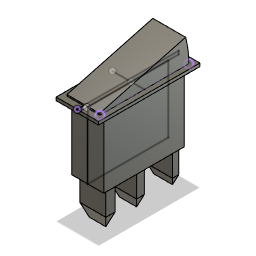
switch v2 (Autodesk Fusion 360 design; units mm, degrees)
Autodesk Fusion 360 part; units mm, degrees
sketch "Sketch1" plane through (0, 0, 0) normal (1, 0, 0) x (0, 0, -1)
  line L0 (0, 0) -> (32.5, 0)
  line L1 (32.5, 0) -> (32.5, -1)
  line L2 (32.5, -1) -> (0, -1)
  line L3 (0, -1) -> (0, 0)
  line L4 (0, -1) -> (3.35, -1) construction
  line L5 (3.35, -1) -> (29.15, -1)
  line L6 (29.15, -1) -> (29.15, -22.4)
  line L7 (29.15, -22.4) -> (3.35, -22.4)
  line L8 (3.35, -22.4) -> (3.35, -1)
  dimension "d1" = 32.5
  dimension "d2" = 1
  dimension "d3" = 3.35
  dimension "d4" = 25.8
  dimension "d5" = 21.4
  constraint horizontal L0
  constraint vertical L1
  constraint horizontal L2
  constraint vertical L3
  constraint coincident L0.start L3.end
  constraint perpendicular L3 L4
  constraint horizontal L5
  constraint vertical L6
  constraint horizontal L7
  constraint vertical L8
  measures "d1" distance of L0.start L0.end
  measures "d2" distance of L0.start L2.end
  measures "d3" distance of L2.end L4.end
  measures "d4" distance of L4.end L5.end
  measures "d5" distance of L4.end L7.end
extrude "Extrude1" add sketch "Sketch1" along normal mid plane 13.6 contours L0 L1 L2 L3 L5 makes body 1
extrude "Extrude2" add sketch "Sketch1" along normal mid plane 10.3 contours L2 L5 L6 L7 L8 bodies 1
sketch "Sketch2" plane through (0, 0, 0) normal (0, 1, 0) x (-1, 0, 0)
  line L0 (6.8, 0) -> (-6.8, 0)
  line L1 (-6.8, 0) -> (-6.8, -32.5)
  line L2 (-6.8, -32.5) -> (6.8, -32.5)
  line L3 (6.8, -32.5) -> (6.8, 0)
  line L4 (6.8, 0) -> (5.25, 0) construction
  line L5 (5.25, 0) -> (5.25, -2) construction
  line L6 (5.25, -2) -> (5.25, -30.5) construction
  line L7 (5.25, -30.5) -> (-5.25, -30.5)
  line L8 (-5.25, -30.5) -> (-5.25, -2)
  line L9 (-5.25, -2) -> (5.25, -2)
  line L10 (5.25, -2) -> (5.25, -30.5)
  dimension "d10" = 1.55
  dimension "d11" = 2
  dimension "d12" = 28.5
  dimension "d13" = 10.5
  constraint coincident L3 L0.start
  constraint perpendicular L3 L4
  constraint coincident L0 L3.end
  constraint perpendicular L0 L5
  constraint perpendicular L2 L6
  constraint horizontal L7
  constraint vertical L8
  constraint horizontal L9
  constraint vertical L10
  measures "d10" distance of L0.start L4.end
  measures "d11" distance of L4.end L5.end
  measures "d12" distance of L5.end L6.end
  measures "d13" distance of L6.end L7.end
sketch "Sketch3" plane through (0, 0, 0) normal (0, 1, 0) x (-1, 0, 0)
  line L0 (-5.25, -30.5) -> (-5.25, -2) construction
  line L1 (-1, -2) -> (-1, -16.25) construction
  line L2 (-5.25, -16.25) -> (5, -16.25)
  dimension "d14" = 28.5
  dimension "d15" = 14.25
  constraint vertical L1
  constraint midpoint L0 L2.start
  constraint perpendicular L0 L2
  measures "d14" distance of L0.start L0.end
  measures "d15" distance of L1.start L1.end
revolve "Revolve1" add sketch "Sketch2" angle 15 about axis through (-6.8, 0, 0) along (1, 0, 0) contours L7 L8 L9 L10 bodies 1
sketch "Sketch4" plane through (0, -22.4, 0) normal (0, -1, 0) x (1, 0, 0)
  line L0 (-5.15, -29.15) -> (5.15, -29.15)
  line L1 (5.15, -29.15) -> (5.15, -3.35)
  line L2 (5.15, -3.35) -> (-5.15, -3.35)
  line L3 (-5.15, -3.35) -> (-5.15, -29.15)
  line L4 (5.15, -4.9865) -> (4.15, -4.9865) construction
  line L5 (5.15, -27.5133) -> (4.15, -27.5133) construction
  line L6 (5.15, -16.25) -> (4.15, -16.25) construction
  line L7 (4.15, -4.9865) -> (-4.15, -4.9865)
  line L8 (-4.15, -4.9865) -> (-4.15, -7.9865)
  line L9 (-4.15, -7.9865) -> (4.15, -7.9865)
  line L10 (4.15, -7.9865) -> (4.15, -4.9865)
  line L11 (-4, -15) -> (4.0078, -15)
  line L12 (4.0078, -15) -> (4.0078, -17.5)
  line L13 (4.0078, -17.5) -> (-4, -17.5)
  line L14 (-4, -17.5) -> (-4, -15)
  line L15 (-4, -15) -> (4.0078, -17.5) construction
  line L16 (4.0078, -15) -> (-4, -17.5) construction
  line L17 (-4, -26.5) -> (4.0078, -26.5)
  line L18 (4.0078, -26.5) -> (4.0078, -28.5266)
  line L19 (4.0078, -28.5266) -> (-4, -28.5266)
  line L20 (-4, -28.5266) -> (-4, -26.5)
  line L21 (-4, -26.5) -> (4.0078, -28.5266) construction
  line L22 (4.0078, -26.5) -> (-4, -28.5266) construction
  point P0 (0.0039, -16.25)
  point P1 (0.0039, -27.5133)
  dimension "d17" = 10.3
  dimension "d18" = 1
  dimension "d19" = 1
  dimension "d20" = 1
  dimension "d21" = 8.3
  dimension "d22" = 3
  constraint coincident L1 L4.start
  constraint perpendicular L1 L4
  constraint coincident L1 L5.start
  constraint perpendicular L1 L5
  constraint midpoint L1 L6.start
  constraint perpendicular L1 L6
  constraint horizontal L7
  constraint vertical L8
  constraint horizontal L9
  constraint vertical L10
  constraint horizontal L11
  constraint perpendicular L11 L12
  constraint parallel L11 L13
  constraint parallel L12 L14
  constraint coincident L15 P0
  constraint coincident L16 P0
  constraint horizontal L17
  constraint perpendicular L17 L18
  constraint parallel L17 L19
  constraint parallel L18 L20
  constraint coincident L21 P1
  constraint coincident L22 P1
  measures "d17" distance of L1.end L2.end
  measures "d18" distance of L4.start L4.end
  measures "d19" distance of L5.start L5.end
  measures "d20" distance of L6.start L6.end
  measures "d21" distance of L4.end L7.end
  measures "d22" distance of L7.end L8.end
extrude "Extrude3" add sketch "Sketch4" along normal blind 8 contours L7 L8 L9 L10 | L11 L12 L13 L14 | L17 L18 L19 L20 bodies 1
extrude "Extrude4" add 3 faces at (-1.3307, -30.4, -27.1755) (-1.3307, -30.4, -15.8333) (-1.3833, -30.4, -5.9865) along direction (0, -1, 0) blind 6 draft -20 on bodies 1 bodies 1
copy_body "Body->Comp1" bodies 1 removing the originals makes body 2 in component "Switch"
component "Switch" placed x (1, 0, 0) y (0, 1, 0) z (0, 0, 1) at (0, 0, 0)
equation "d6 = ( 13.6 / 2 ) * 1 mm"
equation "d8 = ( 10.3 / 2 ) * 1 mm"
equation "d10 = ( ( 13.6 - 10.5 ) / 2 ) * 1 mm"
equation "d12 = 30.500 mm - 2 mm"
equation "d15 = ( 28.5 / 2 ) * 1 mm"
equation "d21 = 10.3 mm - 2 mm"
